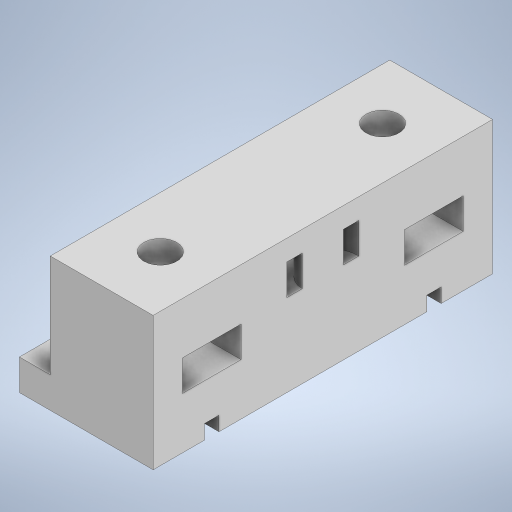
# Autodesk Inventor part: hotend magnet
Saved by Autodesk Inventor 2023.1 (Build 271208000, 208)
## iProperties
Created: 2022-11-07
Part Number: hotend magnet
Material: Generic
Document SubType Name: Modeling
Designer: nicol
Density: 1 g/cm^3
Appearance: Default
Author: nicol
Autodesk Inventor part; units mm, degrees
ref_plane "YZ Plane" through (0, 0, 0) normal (1, 0, 0) x (0, 1, 0)
ref_plane "XZ Plane" through (0, 0, 0) normal (0, 1, 0) x (-1, 0, 0)
sketch "Sketch1" plane through (0, 0, 0) normal (0, 0, 1) x (1, 0, 0)
  line L0 (0, 0) -> (3, 0)
  line L1 (3, 0) -> (3, 10)
  line L2 (3, 10) -> (13, 10)
  line L3 (13, 10) -> (13, -3)
  line L4 (13, -3) -> (0, -3)
  line L5 (0, -3) -> (0, 0)
  dimension "d0" = 10
  dimension "d1" = 3
  dimension "d2" = 3
  dimension "d3" = 10
  constraints: 12 end point, 5 perpendicular, 1 horizontal
  measures "d0" distance of L1.end L2.end
  measures "d1" distance between parallel lines of L5 L1
  measures "d2" distance of L4.end L0.start
  measures "d3" distance of L0.end L1.end
extrude "Extrusion1" add sketch "Sketch1" along normal blind 33
sketch "Sketch2" plane through (0, -3, 0) normal (0, -1, 0) x (1, 0, 0)
  line L0 (13, 0) -> (3, 0) projected
  line L1 (3, 0) -> (3, 33) projected
  line L2 (13, 33) -> (3, 33) projected
  line L3 (13, 0) -> (13, 33) projected
  line L4 (0, 33) -> (13, 33) projected
  line L5 (6.3546, 24.45) -> (4.7091, 27.3)
  line L6 (4.7091, 27.3) -> (6.3546, 30.15)
  line L7 (6.3546, 30.15) -> (9.6454, 30.15)
  line L8 (9.6454, 30.15) -> (11.2909, 27.3) construction
  line L9 (11.2909, 27.3) -> (9.6454, 24.45) construction
  line L10 (9.6454, 24.45) -> (6.3546, 24.45)
  line L11 (6.3546, 2.85) -> (4.7091, 5.7)
  line L12 (4.7091, 5.7) -> (6.3546, 8.55)
  line L13 (6.3546, 8.55) -> (9.6454, 8.55)
  line L14 (9.6454, 8.55) -> (11.2909, 5.7) construction
  line L15 (11.2909, 5.7) -> (9.6454, 2.85) construction
  line L16 (9.6454, 2.85) -> (6.3546, 2.85)
  line L17 (9.6454, 30.15) -> (9.6454, 24.45) construction
  line L18 (9.6454, 24.45) -> (13, 24.45)
  line L19 (13, 24.45) -> (13, 30.15)
  line L20 (13, 30.15) -> (9.6454, 30.15)
  line L21 (9.6454, 8.55) -> (9.6454, 2.85) construction
  line L22 (9.6454, 2.85) -> (13, 2.85)
  line L23 (13, 2.85) -> (13, 8.55)
  line L24 (13, 8.55) -> (9.6454, 8.55)
  line L25 (13, 0) -> (13, 33) projected
  point P0 (0, 0)
  point P1 (8, 27.3)
  point P2 (8, 5.7)
  point P3 (8, 33)
  point P4 (6.5, 33)
  point P5 (8, 27.3)
  point P6 (8, 5.7)
  point P7 (13, 8.55)
  point P8 (13, 30.15)
  dimension "d6" = 21.6
  dimension "d7" = 5.7
  dimension "d8" = 5.7
  dimension "d19" = 5.7
  constraints: 40 end point, 5 parallel, 4 perpendicular, 2 coincident, 2 collinear, 2 midpoint, 2 vertical alignment, 1 equal length, 1 horizontal, 26 other
  measures "d6" distance of point (8, 5.7) point (8, 27.3)
  measures "d7" distance from line of L0 point (8, 5.7)
  measures "d8" vertical distance of point (6.5, 33) point (8, 27.3)
  measures "d19" distance between parallel lines of L7 L10
hole "Hole1" at (8, -3, 27.3) at (8, -3, 5.7) direction (0, 1, 0) diameter 3.2 end through all countersink diameter 6 countersink angle 90
sketch "Sketch3" plane through (0, -3, 0) normal (0, -1, 0) x (1, 0, 0)
  circle A0 centre (8, 27.3) radius 3 projected
  circle A1 centre (8, 5.7) radius 3 projected
  line L0 (0, 0) -> (13, 0) projected
  line L1 (13, 0) -> (13, 33) projected
  line L2 (0, 33) -> (13, 33) projected
  line L3 (0, 0) -> (0, 33) projected
  circle A2 centre (8, 5.7) radius 3 projected
  circle A3 centre (8, 5.7) radius 1.6 projected
  circle A4 centre (8, 27.3) radius 3 projected
  circle A5 centre (8, 27.3) radius 1.6 projected
  line L4 (13, 28) -> (8, 28)
  line L5 (8, 28) -> (8, 26.6)
  line L6 (8, 26.6) -> (13, 26.6)
  line L7 (13, 26.6) -> (13, 28)
  line L8 (13, 6.4) -> (8, 6.4)
  line L9 (8, 6.4) -> (8, 5)
  line L10 (8, 5) -> (13, 5)
  line L11 (13, 5) -> (13, 6.4)
  point P0 (0, 0)
  point P1 (13, 16.5)
  dimension "d16" = 1.4
  constraints: 16 end point, 4 coincident, 4 parallel, 3 midpoint, 2 horizontal, 2 perpendicular, 2 point on line, 1 collinear
  measures "d16" distance between parallel lines of L4 L6
extrude "Extrusion2" cut sketch "Sketch3" against normal blind 1.4 contours A0 L6 A5 L4 | A0 L4 L1 L6 | A5 L6 L5 L4 | L1 L10 A1 L8 | A1 L10 A3 L8 | A3 L10 L9 L8 picked at (10.0575, 27.1414) picked at (8.5333, 27.3) picked at (10.0575, 5.8586) picked at (8.5333, 5.7)
ref_plane "Work Plane1" through (0, 2, 0) normal (0, -1, 0) x (1, 0, 0)
extrude "Extrusion3" cut sketch "Sketch2" against normal blind 3 from surface at -5 contours L22 L16 L11 L12 L13 L24 L3 | L18 L10 L5 L6 L7 L20 L3
sketch "Sketch4" plane through (13, -3, 0) normal (1, 0, 0) x (0, 0, -1)
  line L0 (0, 13) -> (-33, 13) projected
  line L1 (-16.5, 13) -> (-16.5, 0)
  line L2 (-6.4, 0) -> (-26.6, 0) projected
  line L3 (-14.5, 11) -> (-13, 11)
  line L4 (-13, 11) -> (-13, 8)
  line L5 (-13, 8) -> (-14.5, 8)
  line L6 (-14.5, 8) -> (-14.5, 11)
  point P0 (0, 3)
  dimension "d23" = 3
  dimension "d24" = 1.5
  dimension "d25" = 2
  dimension "d26" = 2
  constraints: 10 end point, 2 midpoint, 2 parallel, 1 horizontal, 1 perpendicular, 1 vertical
  measures "d23" distance of L3.end L4.end
  measures "d24" distance of L3.start L3.end
  measures "d25" distance between parallel lines of L1 L6
  measures "d26" distance between parallel lines of L0 L3
revolve "Revolution1" cut sketch "Sketch4" angle 360 about axis through (13, 10, 16.5) along (0, -1, 0)
equation "\"d7\" = d8"
body "Solid1"
